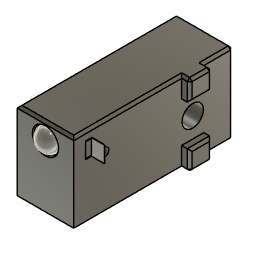
Ball probes (Autodesk Fusion 360 archive; units mm, degrees)
design "Calibration pin 6mm dual ball"
Autodesk Fusion 360 part; units mm, degrees
sketch "Sketch1" plane through (0, 0, 0) normal (0, 1, 0) x (1, 0, 0)
  circle A0 centre (0, 0) radius 3 construction
  circle A1 centre (0, 0) radius 3.3
  line L0 (3.0406, 3.0406) -> (-3.0406, 3.0406) construction
  line L1 (-3.0406, 3.0406) -> (-3.0406, -3.0406) construction
  line L2 (-3.0406, -3.0406) -> (3.0406, -3.0406) construction
  line L3 (3.0406, -3.0406) -> (3.0406, 3.0406) construction
  line L4 (3.0406, 3.0406) -> (-3.0406, -3.0406) construction
  line L5 (-3.0406, 3.0406) -> (3.0406, -3.0406) construction
  circle A2 centre (-3.0406, -3.0406) radius 1.25
  circle A3 centre (3.0406, -3.0406) radius 1.25
  circle A4 centre (3.0406, 3.0406) radius 1.25
  circle A5 centre (-3.0406, 3.0406) radius 1.25
  circle A6 centre (0, 0) radius 3.05 construction
  line L6 (0, 0) -> (0, 8.484) construction
  line L7 (7, -4.1406) -> (-7, -4.1406)
  line L8 (-7, -4.1406) -> (-7, 15.8594)
  line L9 (-7, 15.8594) -> (7, 15.8594)
  line L10 (7, 15.8594) -> (7, -4.1406)
  line L11 (7, -4.1406) -> (-7, 15.8594) construction
  line L12 (-7, -4.1406) -> (7, 15.8594) construction
  circle A7 centre (0, 0) radius 1.25
  point P0 (0, 5.8594)
  dimension "d1" = 6
  dimension "d2" = 6.6
  dimension "d3" = 2.5
  dimension "d4" = 2.5
  dimension "d5" = 2.5
  dimension "d6" = 2.5
  dimension "d7" = 6.1
  dimension "d9" = 1.1
  dimension "d27" = 20
  dimension "d28" = 14
  dimension "d57" = 135
  dimension "d72" = 2.5
  constraint coincident A0.centre A1.centre
  constraint concentric A0 A1
  constraint horizontal L0
  constraint perpendicular L0 L1
  constraint parallel L0 L2
  constraint parallel L1 L3
  constraint coincident L4 A0.centre
  constraint coincident L5 A0.centre
  constraint coincident L1.end L2.start
  constraint coincident L2.end L3.start
  constraint coincident L0.start L3.end
  constraint coincident L0.end L1.start
  constraint tangent A5 A6
  constraint vertical L6
  constraint horizontal L7
  constraint perpendicular L7 L8
  constraint parallel L7 L9
  constraint parallel L8 L10
  constraint coincident L11 P0
  constraint coincident L12 P0
  constraint coincident L6 P0
  constraint concentric A1 A7
  measures "d1" diameter of A0
  measures "d2" diameter of A1
  measures "d3" diameter of A2
  measures "d4" diameter of A3
  measures "d5" diameter of A4
  measures "d6" diameter of A5
  measures "d7" diameter of A6
  measures "d9" distance of L1.end L7
  measures "d27" distance of L7 L9
  measures "d28" distance of L8 L10
  measures "d57" angle of L4 L6
  measures "d72" diameter of A7
extrude "Extrude1" add sketch "Sketch1" along normal blind 20 contours A1 A2 A3 A4 A5 | A1 A2 A3 A4 A5 L7 L8 L9 L10 | A1 A4 | A1 A4 | A1 A3 L7 | A1 A3 | A1 A2 A3 L7 | A1 A5 | A1 A5 | A1 A2 L7 | A1 A2 | A7 makes body 1
ref_plane "WorkPlane1" through (0, 10, -5.8594) normal (-1, 0, 0) x (0, 0, 1)
sketch "Sketch2" plane through (0, 0, 0) normal (-1, 0, 0) x (0, -1, 0)
  line L0 (0, 4.1406) -> (-20, 4.1406)
  line L1 (-20, -15.8594) -> (0, -15.8594)
  line L2 (0, 0) -> (-11.1899, 0)
  circle A0 centre (-1.2, 0) radius 3
  line L3 (0, 0) -> (4.1244, 0)
  line L4 (0, -15.8594) -> (0, 4.1406)
  line L5 (-20, 4.1406) -> (-20, -15.8594)
  circle A1 centre (-1.2, 0) radius 3.2
  line L6 (-19.5, 8.6015) -> (-19.5, -18.3557)
  line L7 (0, -15.8594) -> (0, 4.1406)
  line L8 (-19.5, 4.1406) -> (-39.5, 4.1406)
  line L9 (-39.5, 4.1406) -> (-39.5, -15.8594)
  line L10 (-39.5, -15.8594) -> (-19.5, -15.8594)
  line L11 (-19.5, -15.8594) -> (-19.5, 4.1406)
  line L12 (-29.5, -15.8594) -> (-29.5, 4.1406) construction
  circle A2 centre (-29.5, -5.8594) radius 2.65
  line L13 (-32.25, -15.8594) -> (-26.75, -15.8594)
  line L14 (-26.75, -15.8594) -> (-26.75, -10.8594)
  line L15 (-26.75, -10.8594) -> (-32.25, -10.8594)
  line L16 (-32.25, -10.8594) -> (-32.25, -15.8594)
  line L17 (-32.25, -15.8594) -> (-26.75, -10.8594) construction
  line L18 (-26.75, -15.8594) -> (-32.25, -10.8594) construction
  line L19 (-32.25, 4.1406) -> (-26.75, 4.1406)
  line L20 (-26.75, 4.1406) -> (-26.75, -0.8594)
  line L21 (-26.75, -0.8594) -> (-32.25, -0.8594)
  line L22 (-32.25, -0.8594) -> (-32.25, 4.1406)
  line L23 (-32.25, 4.1406) -> (-26.75, -0.8594) construction
  line L24 (-26.75, 4.1406) -> (-32.25, -0.8594) construction
  circle A3 centre (-29.5, -5.8594) radius 4.5
  circle A4 centre (-7.5, 0) radius 3
  circle A5 centre (-7.5, 0) radius 3.1
  circle A6 centre (-7.5, 0) radius 3.2
  line L25 (-1.2, 3.2) -> (-7.5, 3.2)
  line L26 (-7.5, -3.2) -> (-1.2, -3.2)
  line L27 (-7.5, -3.2) -> (-7.5, 3.2)
  line L28 (-7.5, 3.1) -> (-4.2029, 3.1)
  line L29 (-4.2029, 3.1) -> (-4.2029, 3.2)
  line L30 (-4.2029, 3.2) -> (-7.5, 3.2)
  line L31 (-7.5, 3.2) -> (-7.5, 3.1)
  line L32 (-7.5, -3.1) -> (-3.9603, -3.1)
  line L33 (-3.9603, -3.1) -> (-3.9603, -3.2)
  line L34 (-3.9603, -3.2) -> (-7.5, -3.2)
  line L35 (-7.5, -3.2) -> (-7.5, -3.1)
  point P0 (-29.5, -13.3594)
  point P1 (-29.5, 1.6406)
  dimension "d12" = 6
  dimension "d18" = 6.4
  dimension "d24" = 19.5
  dimension "d25" = 20
  dimension "d26" = 20
  dimension "d31" = 5.3
  dimension "d32" = 5.5
  dimension "d33" = 5
  dimension "d34" = 5.5
  dimension "d35" = 5
  dimension "d49" = 1.2
  dimension "d53" = 9
  dimension "d69" = 6
  dimension "d70" = 6.2
  dimension "d71" = 6.4
  dimension "d76" = 6.3
  constraint coincident L2.start L3.start
  constraint horizontal L2
  constraint coincident L2 A0.centre
  constraint parallel L2 L3
  constraint concentric A0 A1
  constraint perpendicular L0 L6
  constraint horizontal L8
  constraint vertical L9
  constraint horizontal L10
  constraint vertical L11
  constraint coincident L0 L8.start
  constraint coincident L6 L8.start
  constraint midpoint L10 L12.start
  constraint midpoint L8 L12.end
  constraint midpoint L12 A2.centre
  constraint horizontal L13
  constraint perpendicular L13 L14
  constraint parallel L13 L15
  constraint parallel L14 L16
  constraint coincident L17 P0
  constraint coincident L18 P0
  constraint coincident L12 P0
  constraint collinear L10 L13
  constraint horizontal L19
  constraint perpendicular L19 L20
  constraint parallel L19 L21
  constraint parallel L20 L22
  constraint coincident L23 P1
  constraint coincident L24 P1
  constraint coincident L12 P1
  constraint collinear L8 L19
  constraint concentric A2 A3
  constraint coincident L2 A4.centre
  constraint concentric A4 A5
  constraint concentric A4 A6
  constraint coincident A1 L25.start
  constraint coincident A6 L25.end
  constraint horizontal L25
  constraint tangent A1 L25
  constraint coincident A6 L26.start
  constraint coincident A1 L26.end
  constraint tangent A1 L26
  constraint tangent A6 L26
  constraint perpendicular L25 L27
  constraint horizontal L28
  constraint vertical L29
  constraint horizontal L30
  constraint vertical L31
  constraint coincident L25 L29.end
  constraint coincident L27 L28.start
  constraint coincident A5 L28.start
  constraint horizontal L32
  constraint vertical L33
  constraint horizontal L34
  constraint vertical L35
  constraint coincident L26 L33.end
  constraint coincident L27 L32.start
  constraint coincident A5 L32.start
  measures "d12" diameter of A0
  measures "d18" diameter of A1
  measures "d24" distance of L6 L7
  measures "d25" distance of L8.start L8.end
  measures "d26" distance of L8.start L10.end
  measures "d31" diameter of A2
  measures "d32" distance of L14.end L15.end
  measures "d33" distance of L13.end L14.end
  measures "d34" distance of L20.end L21.end
  measures "d35" distance of L19.end L20.end
  measures "d49" distance of A0.centre L7
  measures "d53" diameter of A3
  measures "d69" diameter of A4
  measures "d70" diameter of A5
  measures "d71" diameter of A6
  measures "d76" distance of A0.centre A4.centre
revolve "Revolve1" add sketch "Sketch2" angle 360 about axis through (0, 0, 0) along (0, -1, 0) separate body contours A0 L3 L4 L7 | L2 A0 L4 L7 | L2 A4 L27 | L2 A4 L27 picked at (1.1895, -0.1444) picked at (-2.79, -0.1411) picked at (-6.0894, -1.4106) picked at (-9.4898, -0.1423) makes body 2 at (0.7091, 1.8384, -2.8442) makes body 3 at (0.7091, 8.1384, -2.8442)
revolve "Revolve2" cut sketch "Sketch2" angle 360 about axis through (0, 0, 0) along (0, -1, 0) contours L2 A0 L4 L7 | A0 L3 L4 L7 | A0 L3 L4 A1 L7 | L2 A0 L4 A1 L7 A6 | L2 A1 A6 | A1 A6 L26 L32 L33 | L2 A4 A5 L27 | A1 A5 A6 L32 | L2 A4 L27 | L2 A4 A5 L27 | L2 A4 L27 picked at (-2.79, 0.1411) picked at (1.1895, 0.1444) picked at (0.2699, -2.6845) picked at (-4.2002, -0.6084) picked at (-4.3648, -0.0629) picked at (-4.5262, -0.7199) picked at (-6.0894, -1.4106) picked at (-9.906, -1.8902) picked at (-9.4898, -0.1423) bodies 1
extrude "Extrude3" add sketch "Sketch1" along normal blind 12 contours A1 A4 | A1 A4 | A1 A3 L7 | A1 A3 | A1 A5 | A1 A5 | A1 A2 L7 | A1 A2 bodies 1
extrude "Extrude4" add sketch "Sketch2" against normal up to surface (14 mm away) from surface at 7 contours L5 L8 L9 L10 L14 L15 L16 L20 L21 L22 | L8 L19 L20 L21 L22 | L10 L13 L14 L15 L16 | A3 bodies 1
extrude "Extrude7" cut sketch "Sketch2" along normal blind 12 from surface at 5 contours A3 bodies 1
extrude "Extrude5" add sketch "Sketch2" against normal blind 2 from surface at -7 contours L8 L19 L20 L21 L22 | L10 L13 L14 L15 L16 bodies 1
extrude "Extrude9" cut sketch "Sketch1" along normal blind 46 contours A7 bodies 1
ref_plane "WorkPlane2" through (0, 5.595, 0) normal (0, 0, 1) x (0, 1, 0)
sketch "Sketch4" plane through (0, 0, 0) normal (0, 0, 1) x (1, 0, 0)
  line L0 (7, 26.75) -> (9, 26.75)
  line L1 (9, 26.75) -> (9, 32.25)
  line L2 (9, 32.25) -> (7, 32.25)
  line L3 (7, 32.25) -> (7, 39.5)
  line L4 (7, 39.5) -> (1.25, 39.5)
  line L5 (1.25, 39.5) -> (1.25, 10.3368)
  arc A0 (1.25, 10.3368) -> (3.1, 7.5) centre (0, 7.5) cw
  line L6 (3.2, 3.9603) -> (3.2, 1.2)
  arc A1 (3.2, 1.2) -> (2.9665, 0) centre (0, 1.2) cw
  line L7 (2.9665, 0) -> (7, 0)
  line L8 (7, 0) -> (7, 26.75)
  line L9 (-7, 0) -> (-2.9665, 0)
  arc A2 (-2.9665, 0) -> (-3.2, 1.2) centre (0, 1.2) cw
  line L10 (-3.2, 1.2) -> (-3.2, 3.9603)
  arc A3 (-3.1, 7.5) -> (-1.25, 10.3368) centre (0, 7.5) cw
  line L11 (-1.25, 10.3368) -> (-1.25, 39.5)
  line L12 (-1.25, 39.5) -> (-7, 39.5)
  line L13 (-7, 39.5) -> (-7, 0)
  circle A4 centre (0, 1.2) radius 3
  circle A5 centre (0, 7.5) radius 3
  line L14 (-1.7008, 4.4) -> (10.2095, 4.4)
  line L15 (10.2095, 4.4) -> (10.2095, 4.5)
  line L16 (10.2095, 4.5) -> (-1.7008, 4.5)
  line L17 (-1.7008, 4.5) -> (-1.7008, 4.4)
  line L18 (3.2, 3.6) -> (7, 2.93)
  line L19 (3.2, 3.6) -> (7.1666, 3.6) construction
  line L20 (-1.5847, 4.0489) -> (-1.6847, 4.0489)
  line L21 (-1.6847, 4.0489) -> (-1.6847, 4.1489)
  line L22 (-1.6847, 4.1489) -> (-1.5847, 4.1489)
  line L23 (-1.5847, 4.1489) -> (-1.5847, 4.0489)
  spline S0 degree 5 poles (3.1, 4.4) (2.9118, 4.4) (2.5357, 4.3959) (1.9722, 4.3775) (1.2221, 4.3317) (0.2857, 4.251) (-0.4627, 4.1749) (-1.0238, 4.1135) (-1.3978, 4.0707) (-1.5847, 4.0489) knots 0 0 0 0 0 0 0.2 0.4 0.6 0.8 1 1 1 1 1 1
  spline S1 degree 5 poles (3.1, 4.5) (2.9118, 4.5) (2.5357, 4.4959) (1.9722, 4.4775) (1.2221, 4.4317) (0.2857, 4.351) (-0.4627, 4.2749) (-1.0238, 4.2135) (-1.3978, 4.1707) (-1.5847, 4.1489) knots 0 0 0 0 0 0 0.2 0.4 0.6 0.8 1 1 1 1 1 1
  line L24 (3.1, 7.5) -> (3.1, 3.9603)
  line L25 (3.1, 3.9603) -> (3.2, 3.9603)
  line L26 (-3.2, 3.9603) -> (-3.1, 3.9603)
  line L27 (-3.1, 3.9603) -> (-3.1, 7.5)
  dimension "d85" = 0.1
  dimension "d86" = 10
  dimension "d87" = 0.8
  dimension "d88" = 0.1
  dimension "d89" = 0.1
  constraint horizontal L14
  constraint vertical L15
  constraint horizontal L16
  constraint vertical L17
  constraint horizontal L19
  constraint coincident L6 L18.start
  constraint coincident L8 L18.end
  constraint horizontal L20
  constraint vertical L21
  constraint horizontal L22
  constraint vertical L23
  constraint tangent A5 L16
  constraint coincident L16 S1.start
  constraint coincident L14 S0.start
  constraint coincident S1.start L24
  measures "d85" distance of L14.start L16.end
  measures "d86" angle of L18 L19
  measures "d87" distance of L14 L19
  measures "d88" distance of L20.start L20.end
  measures "d89" distance of L20.start L22.end
extrude "Extrude10" cut sketch "Sketch4" along normal mid plane 4 contours L8 L14 L16 L24 | L6 L8 L14 L18 L24 L25 bodies 1
extrude "Extrude11" add sketch "Sketch4" along normal mid plane 4 separate body contours L8 L14 L15 L16 | L8 L14 L16 L24 | L14 S1 L24 | L14 L23 S0 S1 | L20 L21 L22 L23 makes body 4
extrude "Extrude12" add sketch "Sketch4" along normal mid plane 3.6 separate body contours L6 L8 L14 L18 L24 L25 makes body 5
sketch "Sketch5" plane through (0, 0, 0) normal (-1, 0, 0) x (0, -1, 0)
  circle A0 centre (-29.5, -5.8594) radius 2.65
  line L0 (0, -15.8594) -> (0, -2.9665)
  arc A1 (0, -2.9665) -> (-1.2, -3.2) centre (-1.2, 0) cw
  line L1 (-1.2, -3.2) -> (-3.9603, -3.2)
  arc A2 (-7.5, -3.1) -> (-10.3368, -1.25) centre (-7.5, 0) cw
  line L2 (-10.3368, -1.25) -> (-39.5, -1.25)
  line L3 (-39.5, -1.25) -> (-39.5, -15.8594)
  line L4 (-39.5, -15.8594) -> (0, -15.8594)
  line L5 (0, 2.9665) -> (0, 4.1406)
  line L6 (0, 4.1406) -> (-39.5, 4.1406)
  line L7 (-39.5, 4.1406) -> (-39.5, 1.25)
  line L8 (-39.5, 1.25) -> (-10.3368, 1.25)
  arc A3 (-10.3368, 1.25) -> (-7.5, 3.1) centre (-7.5, 0) cw
  line L9 (-3.9603, 3.2) -> (-1.2, 3.2)
  arc A4 (-1.2, 3.2) -> (0, 2.9665) centre (-1.2, 0) cw
  circle A5 centre (-1.2, 0) radius 3
  circle A6 centre (-7.5, 0) radius 3
  circle A7 centre (-7.7345, -2.7735) radius 1
  line L10 (-3.9603, -3.2) -> (-3.9603, -3.1)
  line L11 (-3.9603, -3.1) -> (-7.5, -3.1)
  line L12 (-7.5, 3.1) -> (-3.9603, 3.1)
  line L13 (-3.9603, 3.1) -> (-3.9603, 3.2)
  dimension "d94" = 2
  measures "d94" diameter of A7
extrude "Extrude13" cut sketch "Sketch5" along normal blind -8.5 and the other way blind -2.5 contours A2 A6 A7 L11 | A2 A7 L11 | A6 A7 picked at (-7.7152, -2.5809) bodies 1
fillet "Fillet2" radius 0.2 1 edges at (-1.0727, 0, -2.7657) on bodies 1
chamfer "Chamfer1" distance 0.6 angle 45 5 faces at (-2.3333, 22.0833, -15.8594) (-2.3333, 22.0833, 4.1406) (0.0311, 39.5, -10.9885) (9, 30.4167, -12.5261) (9, 30.4167, 2.4739) on bodies 1
named bodies: "Main", "Ball", "Ball2", "spring", "Wedge"
